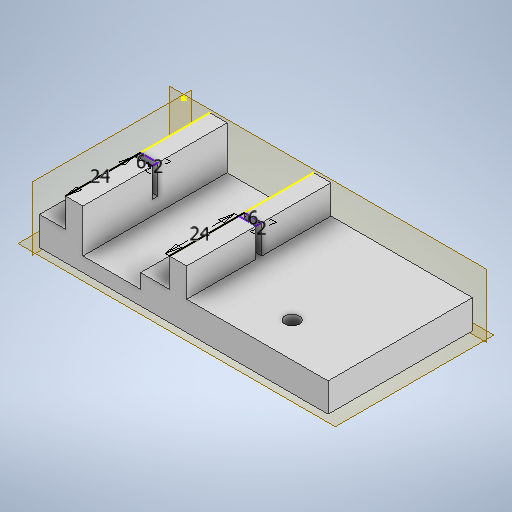
# Autodesk Inventor part: wire_setbaseV2
Saved by Autodesk Inventor 2025.2 (Build 292293000, 293)
## iProperties
Created: 2025-05-08
Part Number: wire_setbaseV2
Material: 一般
Document SubType Name: Modeling
Designer: user
Density: 1 g/cm^3
Appearance: 預設
Author: user
Autodesk Inventor part; units mm, degrees
sketch "草圖1" plane through (0, 0, 0) normal (0, 0, 1) x (1, 0, 0)
  line L0 (0, 0) -> (100, 0)
  line L1 (100, 0) -> (100, 10)
  line L2 (0, 0) -> (0, 10)
  line L3 (0, 10) -> (9, 10)
  line L4 (9, 10) -> (9, 20)
  line L5 (9, 20) -> (15, 20)
  line L6 (15, 20) -> (15, 10)
  line L7 (15, 10) -> (15, 10)
  line L8 (15, 10) -> (15, 5)
  line L9 (15, 5) -> (35, 5)
  line L10 (35, 5) -> (35, 10)
  line L11 (35, 10) -> (45, 10)
  line L12 (45, 10) -> (45, 20)
  line L13 (45, 20) -> (51, 20)
  line L14 (51, 20) -> (51, 10)
  line L15 (51, 10) -> (100, 10)
  dimension "d0" = 100
  dimension "d1" = 10
  dimension "d2" = 10
  dimension "d3" = 9
  dimension "d4" = 10
  dimension "d5" = 6
  dimension "d9" = 5
  dimension "d11" = 20
  dimension "d12" = 10
  dimension "d13" = 6
  constraints: 32 end point, 11 perpendicular, 4 horizontal, 1 point on line, 1 vertical
  measures "d0" distance of L0.start L0.end
  measures "d1" distance of L0.end L1.end
  measures "d2" distance of L0.start L2.end
  measures "d3" distance of L2.end L3.end
  measures "d4" distance of L3.end L4.end
  measures "d5" distance of L4.end L5.end
  measures "d9" distance of L7.end L8.end
  measures "d11" distance of L8.end L9.end
  measures "d12" distance of L10.end L11.end
  measures "d13" distance of L12.end L13.end
extrude "擠出1" add sketch "草圖1" along normal blind 50
sketch "草圖2" plane through (9, 20, 0) normal (0, 1, 0) x (1, 0, 0)
  line L0 (0, 0) -> (0, -50) projected
  line L1 (0, -50) -> (0, -26)
  line L2 (6, -26) -> (6, -24)
  line L3 (0, -26) -> (0, -24)
  line L4 (36, 0) -> (36, -50) projected
  line L5 (36, -50) -> (36, -26)
  line L6 (36, -26) -> (42, -26)
  line L7 (42, -26) -> (42, -24)
  line L8 (42, -24) -> (36, -24)
  line L9 (36, -26) -> (36, -24)
  line L10 (0, -26) -> (6, -26)
  line L11 (6, -24) -> (0, -24)
  line L12 (0, -26) -> (0, -24)
  point P0 (-9, 0)
  dimension "d16" = 24
  dimension "d17" = 2
  dimension "d18" = 24
  dimension "d19" = 6
  dimension "d22" = 6
  dimension "d27" = 2
  constraints: 22 end point, 4 point on line, 3 perpendicular, 2 collinear, 1 parallel
  measures "d16" distance of L0.end L1.end
  measures "d17" distance of L2.start L2.end
  measures "d18" distance of L4.end L5.end
  measures "d19" distance of L5.end L6.end
  measures "d22" distance of L1.end L2.start
  measures "d27" distance of L6.end L7.end
extrude "擠出2" cut sketch "草圖2" against normal up to surface (10 mm away) contours L8 L7 L6 L4
extrude "擠出3" cut sketch "草圖2" against normal up to surface (10 mm away) contours L11 L2 L10 L0
sketch "草圖4" plane through (0, 0, 0) normal (0, 1, 0) x (-1, 0, 0)
  line L0 (0, 50) -> (-100, 50) projected
  line L1 (-100, 50) -> (-100, 38)
  line L2 (-100, 0) -> (-100, 50) projected
  line L3 (-100, 38) -> (-75.5, 38)
  line L4 (-51, 26) -> (-51, 50) projected
  line L5 (0, 50) -> (0, 38)
  line L6 (0, 0) -> (0, 50) projected
  line L7 (0, 38) -> (-4.5, 38)
  dimension "d56" = 12
  dimension "d57" = 24.5
  dimension "d58" = 12
  dimension "d59" = 4.5
  constraints: 8 end point, 2 perpendicular, 2 point on line
  measures "d56" distance of L0.end L1.end
  measures "d57" distance of L1.end L3.end
  measures "d58" distance of L0.start L5.end
  measures "d59" distance of L5.end L7.end
hole "孔3" at (75.5, 0, 38) at (4.5, 0, 38) direction (0, 1, 0) diameter 5 end through all
